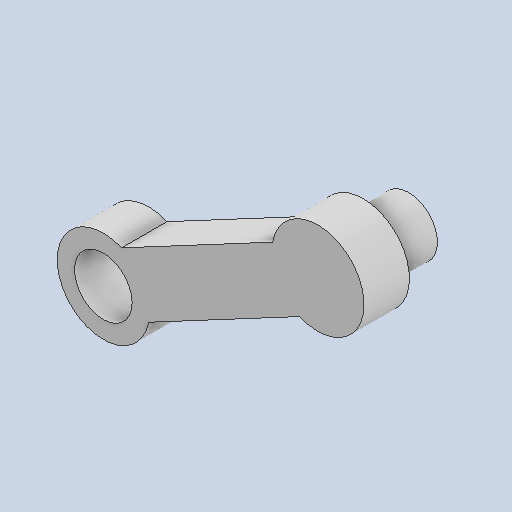
# Autodesk Inventor part: Component32
Saved by Autodesk Inventor 2022 (Build 260153000, 153)
## iProperties
Created: 2022-01-29
Part Number: Component32
Material: Generic
Document SubType Name: Modeling
Designer: Administrator
Density: 1 g/cm^3
Appearance: Default
Title: Component32
Author: Administrator
Autodesk Inventor part; units mm, degrees
ref_plane "YZ Plane" through (0, 0, 0) normal (1, 0, 0) x (0, 1, 0)
ref_plane "XZ Plane" through (0, 0, 0) normal (0, 1, 0) x (-1, 0, 0)
ref_plane "XY Plane" through (0, 0, 0) normal (0, 0, 1) x (1, 0, 0)
sketch "Sketch2" plane through (0, 0, 0) normal (0, 0, 1) x (1, 0, 0)
  line L0 (144.6424, 19.1617) -> (128.0034, 10.2983)
  arc A0 (125.0179, 15.9027) -> (128.0034, 10.2983) centre (123.0107, 11.2361) ccw
  line L1 (125.0179, 15.9027) -> (141.6569, 24.7662)
  arc A1 (144.6424, 19.1617) -> (141.6569, 24.7662) centre (146.6496, 23.8284) ccw
  circle A2 centre (146.6496, 23.8284) radius 3.175
  circle A3 centre (146.6496, 23.8284) radius 3.175
  circle A4 centre (146.6496, 23.8284) radius 5.08
  line L2 (125.0179, 15.9027) -> (141.6569, 24.7662)
  line L3 (141.6569, 24.7662) -> (125.0179, 15.9027)
  line L4 (144.6424, 19.1617) -> (128.0034, 10.2983)
  line L5 (144.6424, 19.1617) -> (128.0034, 10.2983)
  circle A5 centre (123.0107, 11.2361) radius 5.08
  arc A6 (125.0179, 15.9027) -> (128.0034, 10.2983) centre (123.0107, 11.2361) ccw
  circle A7 centre (123.0107, 11.2361) radius 3.175
  circle A8 centre (123.0107, 11.2361) radius 3.175
  circle A9 centre (123.0107, 11.2361) radius 3.175
  point P0 (0, 0)
  constraints: 12 end point, 10 centre point, 6 point on circle, 5 coincident, 2 collinear
extrude "Extrusion3" add sketch "Sketch2" along normal blind 5 contours A4 A1 | L0 A5 L1 A4 | A0 A5 | A2
extrude "Extrusion4" add sketch "Sketch2" against normal blind 5 contours A2
body "Solid2"
